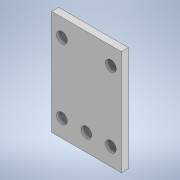
# Autodesk Inventor part: 指支え
Saved by Autodesk Inventor 2022 (Build 260153070, 153G)
## iProperties
Created: 2022-10-10
Part Number: 指支え
Material: 一般
Document SubType Name: Modeling
Designer: hirok
Density: 1 g/cm^3
Appearance: 既定
Author: hirok
Autodesk Inventor part; units mm, degrees
ref_plane "YZ Plane" through (0, 0, 0) normal (1, 0, 0) x (0, 1, 0)
ref_plane "XZ Plane" through (0, 0, 0) normal (0, 1, 0) x (-1, 0, 0)
ref_plane "XY Plane" through (0, 0, 0) normal (0, 0, 1) x (1, 0, 0)
sketch "スケッチ1" plane through (0, 0, 0) normal (0, 0, 1) x (1, 0, 0)
  line L0 (0, 0) -> (20, 0)
  line L1 (20, 0) -> (20, 30)
  line L2 (20, 30) -> (0, 30)
  line L3 (0, 30) -> (0, 0)
  dimension "d0" = 30
  dimension "d1" = 20
  constraints: 8 end point, 2 parallel, 1 horizontal, 1 perpendicular
  measures "d0" distance of L0.end L1.end
  measures "d1" distance of L1.end L2.end
extrude "押し出し1" add sketch "スケッチ1" along normal blind 2
sketch "スケッチ4" plane through (0, 0, 2) normal (0, 0, 1) x (1, 0, 0)
  line L0 (20, 30) -> (0, 30) projected
  line L1 (10, 30) -> (10, 0)
  line L2 (0, 0) -> (20, 0) projected
  point P0 (3, 5)
  point P1 (3, 25)
  point P2 (17, 5)
  point P3 (17, 25)
  dimension "d23" = 7
  dimension "d24" = 7
  dimension "d25" = 20
  dimension "d26" = 5
  constraints: 2 end point, 2 midpoint, 2 symmetric about line
  measures "d23" distance from line of L1 point (3, 5)
  measures "d24" distance from line of L1 point (3, 25)
  measures "d25" distance of point (3, 25) point (3, 5)
  measures "d26" distance from line of L2 point (3, 5)
hole "穴3" at (3, 5, 2) at (3, 25, 2) at (17, 25, 2) at (17, 5, 2) direction (0, 0, -1) diameter 3 end through all
sketch "スケッチ5" plane through (0, 0, 2) normal (0, 0, 1) x (1, 0, 0)
  line L0 (0, 0) -> (20, 0) projected
  point P0 (10, 5)
  dimension "d34" = 5
  measures "d34" distance from line of L0 point (10, 5)
hole "穴4" at (10, 5, 2) direction (0, 0, -1) diameter 3 end through all
